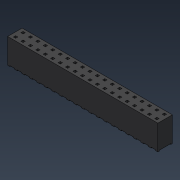
# Autodesk Inventor part: ESQ-120-33-T-D_socket
Saved by Autodesk Inventor 2022.1 (Build 261234020, 234B)
## iProperties
Created: 2017-11-11
Part Number: ESQ-120-33-T-D_socket
Catalog Web Link: www.cadenas.de
Description: ESQ Series Socket-ESQ Series - (2,54 mm) .100'' Elevated Socket
Vendor: SAMTEC
Document SubType Name: Modeling
Designer: psAdmin
Manufacturer: SAMTEC
Mass: 1.93212 g
Surface Area: 23.6719 cm^2
Volume: 1.93212 cm^3
Density: 1 g/cm^3
Material: Allgemein
Appearance: PSOLRGB-127-127-127
Category: PARTsolutions
Company: SAMTEC
PSOL_IDENT_0: {$CADENAS_DATA\23d-libs\samtec\modelling\esq\parts\esq_socket.prj},224 {VTYP=3D},{NB=ESQ-120-33-T-D_
PSOL_IDENT_1: socket},{LINA=ESQ-120-33-T-D_socket},{NN=ESQ Series Socket},{DATE=05.05.2016 11:37:34},{GEOMDATE=05.
PSOL_IDENT_2: 05.2016 11:37:00},{VERSION=},{LINEID=10},{LINESUBID=-1},{WBVAR=POS,LS,PLOPT,ROW,LLOPT,POLOPT}  {NB=E
PSOL_IDENT_3: SQ-120-33-T-D_socket},{LINA=ESQ-120-33-T-D_socket},{KT=DUMMY},{PN=ESQ-120-33-T-D},{SERIES=ESQ},{POS=
PSOL_IDENT_4: 20},{POSN=20},{POSALG=  '01','-01','02','-02','03','-03','04','-04','05','-05','06','-06','07','-07'
PSOL_IDENT_5: ,'08','-08','09','-09','10','-10','11','-11','12','-12','13','-13','14','-14','15','-15','16','-16','
PSOL_IDENT_6: 17','-17','18','-18','19','-19','20','-20','21','-21','22','-22','23','-23','24','-24','25','-25','2
PSOL_IDENT_7: 6','-26','27','-27','28','-28','29','-29','30','-30','31','-31','32','-32','33','-33','34','-34','35'
PSOL_IDENT_8: ,'-35','36','-36'  },{POSPN=20},{LS=33},{PLOPT=T},{PLOPTALG= 'G','-G = 20micro\" Selective Gold in C
PSOL_IDENT_9: ontact Area, 3micro\" Selective Gold on Tail.','T','-T = Matte Tin on Entire Pin.','S','-S =  30micr
PSOL_IDENT_10: o\" Selective Gold in Contact Area, Matte Tin on Tail.','H','-H = 30micro\" Selective Gold in Contac
PSOL_IDENT_11: t Area, 3micro\" Selective Gold on Tail.','F','-F = 3micro\" Selective Gold in Contact Area, Matte T
PSOL_IDENT_12: in on Tail.','E','-E = 50micro\" Selective Gold in Contact Area, 3micro\" Selective Gold on Tail.','
PSOL_IDENT_13: L','-L = 10micro\" Selective Gold in Contact Area, Matte Tin on Tail.' },{ROW=D},{ROWPN=-D},{ROWALG=
PSOL_IDENT_14: 'S','-S = Single Row','D','-D = Double Row','T','-T = Triple Row' },{ROWN=2},{LLOPT=},{LLOPTALG= ''
PSOL_IDENT_15: ,'Not Selected','LL','-LL = Locking Lead' },{LLOPTPN=},{POLOPT=},{POLOPTPN=},{POLOPTMAX=480},{POLOPT
PSOL_IDENT_16: MAX2='001','001','002','002','003','003','004','004','005','005','006','006','007','007','008','008'
PSOL_IDENT_17: ,'009','009','010','010','011','011','012','012','013','013','014','014','015','015','016','016','01
PSOL_IDENT_18: 7','017','018','018','019','019','020','020','021','021','022','022','023','023','024','024','025','
PSOL_IDENT_19: 025','026','026','027','027','028','028','029','029','030','030','031','031','032','032','033','033'
PSOL_IDENT_20: ,'034','034','035','035','036','036','037','037','038','038','039','039','040','040'},{POLOPTALG= ''
PSOL_IDENT_21: ,'Not Selected','001','001','002','002','003','003','004','004','005','005','006','006','007','007','
PSOL_IDENT_22: 008','008','009','009','010','010','011','011','012','012','013','013','014','014','015','015','016'
PSOL_IDENT_23: ,'016','017','017','018','018','019','019','020','020','021','021','022','022','023','023','024','02
PSOL_IDENT_24: 4','025','025','026','026','027','027','028','028','029','029','030','030','031','031','032','032','
PSOL_IDENT_25: 033','033','034','034','035','035','036','036','037','037','038','038','039','039','040','040'},{POL
PSOL_IDENT_26: ARIZE='001','001','002','002','003','003','004','004','005','005','006','006','007','007','008','008'
PSOL_IDENT_27: ,'009','009','010','010','011','011','012','012','013','013','014','014','015','015','016','016','01
PSOL_IDENT_28: 7','017','018','018','019','019','020','020','021','021','022','022','023','023','024','024','025','
PSOL_IDENT_29: 025','026','026','027','027','028','028','029','029','030','030','031','031','032','032','033','033'
PSOL_IDENT_30: ,'034','034','035','035','036','036','037','037','038','038','039','039','040','040','041','041','04
PSOL_IDENT_31: 2','042','043','043','044','044','045','045','046','046','047','047','048','048','049','049','050','
PSOL_IDENT_32: 050','051','051','052','052','053','053','054','054','055','055','056','056','057','057','058','058'
PSOL_IDENT_33: ,'059','059','060','060','061','061','062','062','063','063','064','064','065','065','066','066','06
PSOL_IDENT_34: 7','067','068','068','069','069','070','070','071','071','072','072','073','073','074','074','075','
PSOL_IDENT_35: 075','076','076','077','077','078','078','079','079','080','080','081','081','082','082','083','083'
PSOL_IDENT_36: ,'084','084','085','085','086','086','087','087','088','088','089','089','090','090','091','091','09
PSOL_IDENT_37: 2','092','093','093','094','094','095','095','096','096','097','097','098','098','099','099','100','
PSOL_IDENT_38: 100','101','101','102','102','103','103','104','104','105','105','106','106','107','107','108','108'
PSOL_IDENT_39: ,'109','109','110','110','111','111','112','112','113','113','114','114','115','115','116','116','11
PSOL_IDENT_40: 7','117','118','118','119','119','120','120','121','121','122','122','123','123','124','124','125','
PSOL_IDENT_41: 125','126','126','127','127','128','128','129','129','130','130','131','131','132','132','133','133'
PSOL_IDENT_42: ,'134','134','135','135','136','136','137','137','138','138','139','139','140','140','141','141','14
PSOL_IDENT_43: 2','142','143','143','144','144','145','145','146','146','147','147','148','148','149','149','150','
PSOL_IDENT_44: 150','151','151','152','152','153','153','154','154','155','155','156','156','157','157','158','158'
PSOL_IDENT_45: ,'159','159','160','160','161','161','162','162','163','163','164','164','165','165','166','166','16
PSOL_IDENT_46: 7','167','168','168','169','169','170','170','171','171','172','172','173','173','174','174','175','
PSOL_IDENT_47: 175','176','176','177','177','178','178','179','179','180','180','181','181','182','182','183','183'
PSOL_IDENT_48: ,'184','184','185','185','186','186','187','187','188','188','189','189','190','190','191','191','19
PSOL_IDENT_49: 2','192','193','193','194','194','195','195','196','196','197','197','198','198','199','199','200','
PSOL_IDENT_50: 200','201','201','202','202','203','203','204','204','205','205','206','206','207','207','208','208'
PSOL_IDENT_51: ,'209','209','210','210','211','211','212','212','213','213','214','214','215','215','216','216','21
PSOL_IDENT_52: 7','217','218','218','219','219','220','220','221','221','222','222','223','223','224','224','225','
PSOL_IDENT_53: 225','226','226','227','227','228','228','229','229','230','230','231','231','232','232','233','233'
PSOL_IDENT_54: ,'234','234','235','235','236','236','237','237','238','238','239','239','240','240','241','241','24
PSOL_IDENT_55: 2','242','243','243','244','244','245','245','246','246','247','247','248','248','249','249','250','
PSOL_IDENT_56: 250','251','251','252','252','253','253','254','254','255','255','256','256','257','257','258','258'
PSOL_IDENT_57: ,'259','259','260','260','261','261','262','262','263','263','264','264','265','265','266','266','26
PSOL_IDENT_58: 7','267','268','268','269','269','270','270','271','271','272','272','273','273','274','274','275','
PSOL_IDENT_59: 275','276','276','277','277','278','278','279','279','280','280','281','281','282','282','283','283'
PSOL_IDENT_60: ,'284','284','285','285','286','286','287','287','288','288','289','289','290','290','291','291','29
PSOL_IDENT_61: 2','292','293','293','294','294','295','295','296','296','297','297','298','298','299','299','300','
PSOL_IDENT_62: 300'},{POLARIZEX=0.00000},{POLARIZEY=0.00000},{POLARIZEN=0},{EVEN=0},{A=0.195},{A3DB=0.33500},{B=0.0
PSOL_IDENT_63: 9000},{C=0.635},{D=0.725},{E=0.000},{W=2.02000},{ONES=0}
NN: ESQ Series Socket
NT: ESQ Series - (2,54 mm) .100'' Elevated Socket
NB: ESQ-120-33-T-D_socket
NBSYN: $PN._socket
LINA: ESQ-120-33-T-D_socket
PN: ESQ-120-33-T-D
SERIES: ESQ
POS: -20
LS: -33
PLOPT: -T = Matte Tin on Entire Pin.
ROW: -D = Double Row
LLOPT: Not Selected
POLOPT: Not Selected
A: 0.195
SUPPLIER: SAMTEC
ARTICLENO: ESQ-120-33-T-D_socket
BOMINFO: ESQ-120-33-T-D_socket
CREATOR: CADENAS GmbH
Title: ESQ-120-33-T-D_socket
Author: Cadenas PARTsolutions
Comments: ESQ Series - (2,54 mm) .100'' Elevated Socket
Autodesk Inventor part; units mm, degrees
sketch "Sketch_1" plane through (0, 0, 0) normal (0, 1, 0) x (-1, 0, 0)
  line L0 (0, -2.4765) -> (0, 2.4765)
  line L1 (0, 2.4765) -> (-51.308, 2.4765)
  line L2 (-51.308, 2.4765) -> (-51.308, -2.4765)
  line L3 (-51.308, -2.4765) -> (0, -2.4765)
  line L4 (-49.403, 0.889) -> (-49.403, 1.651)
  line L5 (-49.403, 1.651) -> (-50.165, 1.651)
  line L6 (-50.165, 1.651) -> (-50.165, 0.889)
  line L7 (-50.165, 0.889) -> (-49.403, 0.889)
  line L8 (-49.403, -1.651) -> (-49.403, -0.889)
  line L9 (-49.403, -0.889) -> (-50.165, -0.889)
  line L10 (-50.165, -0.889) -> (-50.165, -1.651)
  line L11 (-50.165, -1.651) -> (-49.403, -1.651)
  line L12 (-46.863, 0.889) -> (-46.863, 1.651)
  line L13 (-46.863, 1.651) -> (-47.625, 1.651)
  line L14 (-47.625, 1.651) -> (-47.625, 0.889)
  line L15 (-47.625, 0.889) -> (-46.863, 0.889)
  line L16 (-46.863, -1.651) -> (-46.863, -0.889)
  line L17 (-46.863, -0.889) -> (-47.625, -0.889)
  line L18 (-47.625, -0.889) -> (-47.625, -1.651)
  line L19 (-47.625, -1.651) -> (-46.863, -1.651)
  line L20 (-44.323, 0.889) -> (-44.323, 1.651)
  line L21 (-44.323, 1.651) -> (-45.085, 1.651)
  line L22 (-45.085, 1.651) -> (-45.085, 0.889)
  line L23 (-45.085, 0.889) -> (-44.323, 0.889)
  line L24 (-44.323, -1.651) -> (-44.323, -0.889)
  line L25 (-44.323, -0.889) -> (-45.085, -0.889)
  line L26 (-45.085, -0.889) -> (-45.085, -1.651)
  line L27 (-45.085, -1.651) -> (-44.323, -1.651)
  line L28 (-41.783, 0.889) -> (-41.783, 1.651)
  line L29 (-41.783, 1.651) -> (-42.545, 1.651)
  line L30 (-42.545, 1.651) -> (-42.545, 0.889)
  line L31 (-42.545, 0.889) -> (-41.783, 0.889)
  line L32 (-41.783, -1.651) -> (-41.783, -0.889)
  line L33 (-41.783, -0.889) -> (-42.545, -0.889)
  line L34 (-42.545, -0.889) -> (-42.545, -1.651)
  line L35 (-42.545, -1.651) -> (-41.783, -1.651)
  line L36 (-39.243, 0.889) -> (-39.243, 1.651)
  line L37 (-39.243, 1.651) -> (-40.005, 1.651)
  line L38 (-40.005, 1.651) -> (-40.005, 0.889)
  line L39 (-40.005, 0.889) -> (-39.243, 0.889)
  line L40 (-39.243, -1.651) -> (-39.243, -0.889)
  line L41 (-39.243, -0.889) -> (-40.005, -0.889)
  line L42 (-40.005, -0.889) -> (-40.005, -1.651)
  line L43 (-40.005, -1.651) -> (-39.243, -1.651)
  line L44 (-36.703, 0.889) -> (-36.703, 1.651)
  line L45 (-36.703, 1.651) -> (-37.465, 1.651)
  line L46 (-37.465, 1.651) -> (-37.465, 0.889)
  line L47 (-37.465, 0.889) -> (-36.703, 0.889)
  line L48 (-36.703, -1.651) -> (-36.703, -0.889)
  line L49 (-36.703, -0.889) -> (-37.465, -0.889)
  line L50 (-37.465, -0.889) -> (-37.465, -1.651)
  line L51 (-37.465, -1.651) -> (-36.703, -1.651)
  line L52 (-34.163, 0.889) -> (-34.163, 1.651)
  line L53 (-34.163, 1.651) -> (-34.925, 1.651)
  line L54 (-34.925, 1.651) -> (-34.925, 0.889)
  line L55 (-34.925, 0.889) -> (-34.163, 0.889)
  line L56 (-34.163, -1.651) -> (-34.163, -0.889)
  line L57 (-34.163, -0.889) -> (-34.925, -0.889)
  line L58 (-34.925, -0.889) -> (-34.925, -1.651)
  line L59 (-34.925, -1.651) -> (-34.163, -1.651)
  line L60 (-31.623, 0.889) -> (-31.623, 1.651)
  line L61 (-31.623, 1.651) -> (-32.385, 1.651)
  line L62 (-32.385, 1.651) -> (-32.385, 0.889)
  line L63 (-32.385, 0.889) -> (-31.623, 0.889)
  line L64 (-31.623, -1.651) -> (-31.623, -0.889)
  line L65 (-31.623, -0.889) -> (-32.385, -0.889)
  line L66 (-32.385, -0.889) -> (-32.385, -1.651)
  line L67 (-32.385, -1.651) -> (-31.623, -1.651)
  line L68 (-29.083, 0.889) -> (-29.083, 1.651)
  line L69 (-29.083, 1.651) -> (-29.845, 1.651)
  line L70 (-29.845, 1.651) -> (-29.845, 0.889)
  line L71 (-29.845, 0.889) -> (-29.083, 0.889)
  line L72 (-29.083, -1.651) -> (-29.083, -0.889)
  line L73 (-29.083, -0.889) -> (-29.845, -0.889)
  line L74 (-29.845, -0.889) -> (-29.845, -1.651)
  line L75 (-29.845, -1.651) -> (-29.083, -1.651)
  line L76 (-26.543, 0.889) -> (-26.543, 1.651)
  line L77 (-26.543, 1.651) -> (-27.305, 1.651)
  line L78 (-27.305, 1.651) -> (-27.305, 0.889)
  line L79 (-27.305, 0.889) -> (-26.543, 0.889)
  line L80 (-26.543, -1.651) -> (-26.543, -0.889)
  line L81 (-26.543, -0.889) -> (-27.305, -0.889)
  line L82 (-27.305, -0.889) -> (-27.305, -1.651)
  line L83 (-27.305, -1.651) -> (-26.543, -1.651)
  line L84 (-24.003, 0.889) -> (-24.003, 1.651)
  line L85 (-24.003, 1.651) -> (-24.765, 1.651)
  line L86 (-24.765, 1.651) -> (-24.765, 0.889)
  line L87 (-24.765, 0.889) -> (-24.003, 0.889)
  line L88 (-24.003, -1.651) -> (-24.003, -0.889)
  line L89 (-24.003, -0.889) -> (-24.765, -0.889)
  line L90 (-24.765, -0.889) -> (-24.765, -1.651)
  line L91 (-24.765, -1.651) -> (-24.003, -1.651)
  line L92 (-21.463, 0.889) -> (-21.463, 1.651)
  line L93 (-21.463, 1.651) -> (-22.225, 1.651)
  line L94 (-22.225, 1.651) -> (-22.225, 0.889)
  line L95 (-22.225, 0.889) -> (-21.463, 0.889)
  line L96 (-21.463, -1.651) -> (-21.463, -0.889)
  line L97 (-21.463, -0.889) -> (-22.225, -0.889)
  line L98 (-22.225, -0.889) -> (-22.225, -1.651)
  line L99 (-22.225, -1.651) -> (-21.463, -1.651)
  line L100 (-18.923, 0.889) -> (-18.923, 1.651)
  line L101 (-18.923, 1.651) -> (-19.685, 1.651)
  line L102 (-19.685, 1.651) -> (-19.685, 0.889)
  line L103 (-19.685, 0.889) -> (-18.923, 0.889)
  line L104 (-18.923, -1.651) -> (-18.923, -0.889)
  line L105 (-18.923, -0.889) -> (-19.685, -0.889)
  line L106 (-19.685, -0.889) -> (-19.685, -1.651)
  line L107 (-19.685, -1.651) -> (-18.923, -1.651)
  line L108 (-16.383, 0.889) -> (-16.383, 1.651)
  line L109 (-16.383, 1.651) -> (-17.145, 1.651)
  line L110 (-17.145, 1.651) -> (-17.145, 0.889)
  line L111 (-17.145, 0.889) -> (-16.383, 0.889)
  line L112 (-16.383, -1.651) -> (-16.383, -0.889)
  line L113 (-16.383, -0.889) -> (-17.145, -0.889)
  line L114 (-17.145, -0.889) -> (-17.145, -1.651)
  line L115 (-17.145, -1.651) -> (-16.383, -1.651)
  line L116 (-13.843, 0.889) -> (-13.843, 1.651)
  line L117 (-13.843, 1.651) -> (-14.605, 1.651)
  line L118 (-14.605, 1.651) -> (-14.605, 0.889)
  line L119 (-14.605, 0.889) -> (-13.843, 0.889)
  line L120 (-13.843, -1.651) -> (-13.843, -0.889)
  line L121 (-13.843, -0.889) -> (-14.605, -0.889)
  line L122 (-14.605, -0.889) -> (-14.605, -1.651)
  line L123 (-14.605, -1.651) -> (-13.843, -1.651)
  line L124 (-11.303, 0.889) -> (-11.303, 1.651)
  line L125 (-11.303, 1.651) -> (-12.065, 1.651)
  line L126 (-12.065, 1.651) -> (-12.065, 0.889)
  line L127 (-12.065, 0.889) -> (-11.303, 0.889)
  line L128 (-11.303, -1.651) -> (-11.303, -0.889)
  line L129 (-11.303, -0.889) -> (-12.065, -0.889)
  line L130 (-12.065, -0.889) -> (-12.065, -1.651)
  line L131 (-12.065, -1.651) -> (-11.303, -1.651)
  line L132 (-8.763, 0.889) -> (-8.763, 1.651)
  line L133 (-8.763, 1.651) -> (-9.525, 1.651)
  line L134 (-9.525, 1.651) -> (-9.525, 0.889)
  line L135 (-9.525, 0.889) -> (-8.763, 0.889)
  line L136 (-8.763, -1.651) -> (-8.763, -0.889)
  line L137 (-8.763, -0.889) -> (-9.525, -0.889)
  line L138 (-9.525, -0.889) -> (-9.525, -1.651)
  line L139 (-9.525, -1.651) -> (-8.763, -1.651)
  line L140 (-6.223, 0.889) -> (-6.223, 1.651)
  line L141 (-6.223, 1.651) -> (-6.985, 1.651)
  line L142 (-6.985, 1.651) -> (-6.985, 0.889)
  line L143 (-6.985, 0.889) -> (-6.223, 0.889)
  line L144 (-6.223, -1.651) -> (-6.223, -0.889)
  line L145 (-6.223, -0.889) -> (-6.985, -0.889)
  line L146 (-6.985, -0.889) -> (-6.985, -1.651)
  line L147 (-6.985, -1.651) -> (-6.223, -1.651)
  line L148 (-3.683, 0.889) -> (-3.683, 1.651)
  line L149 (-3.683, 1.651) -> (-4.445, 1.651)
  line L150 (-4.445, 1.651) -> (-4.445, 0.889)
  line L151 (-4.445, 0.889) -> (-3.683, 0.889)
  line L152 (-3.683, -1.651) -> (-3.683, -0.889)
  line L153 (-3.683, -0.889) -> (-4.445, -0.889)
  line L154 (-4.445, -0.889) -> (-4.445, -1.651)
  line L155 (-4.445, -1.651) -> (-3.683, -1.651)
  line L156 (-1.143, 0.889) -> (-1.143, 1.651)
  line L157 (-1.143, 1.651) -> (-1.905, 1.651)
  line L158 (-1.905, 1.651) -> (-1.905, 0.889)
  line L159 (-1.905, 0.889) -> (-1.143, 0.889)
  line L160 (-1.143, -1.651) -> (-1.143, -0.889)
  line L161 (-1.143, -0.889) -> (-1.905, -0.889)
  line L162 (-1.905, -0.889) -> (-1.905, -1.651)
  line L163 (-1.905, -1.651) -> (-1.143, -1.651)
  constraints: 328 end point
extrude "Extrusion1" add sketch "Sketch_1" along normal blind 8.509
sketch "Sketch_2" plane through (0, 0, 0) normal (0, 1, 0) x (-1, 0, 0)
  line L0 (0, -2.4765) -> (0, 2.4765)
  line L1 (0, 2.4765) -> (-51.308, 2.4765)
  line L2 (-51.308, 2.4765) -> (-51.308, -2.4765)
  line L3 (-51.308, -2.4765) -> (0, -2.4765)
  constraints: 8 end point
extrude "Extrusion2" add sketch "Sketch_2" along normal blind 1.143
sketch "Sketch_9" plane through (0, 0, 0) normal (1, 0, 0) x (0, 1, 0)
  line L0 (0.254, 1.9685) -> (0, 1.9685)
  line L1 (0, 1.9685) -> (0, -1.9685)
  line L2 (0, -1.9685) -> (0.254, -1.9685)
  line L3 (0.254, -1.9685) -> (0.254, 1.9685)
  constraints: 8 end point
extrude "Extrusion3" cut sketch "Sketch_9" along normal blind 51.308
sketch "Sketch_11" plane through (0, 0, 0) normal (0, 0, 1) x (1, 0, 0)
  line L0 (0.254, 0) -> (0.254, -1.27)
  line L1 (0.254, -1.27) -> (51.562, -1.27)
  line L2 (51.562, -1.27) -> (51.562, 0)
  line L3 (51.562, 0) -> (50.546, 0)
  line L4 (50.546, 0) -> (50.546, 0.254)
  line L5 (50.546, 0.254) -> (49.022, 0.254)
  line L6 (49.022, 0.254) -> (49.022, 0)
  line L7 (49.022, 0) -> (48.006, 0)
  line L8 (48.006, 0) -> (48.006, 0.254)
  line L9 (48.006, 0.254) -> (46.482, 0.254)
  line L10 (46.482, 0.254) -> (46.482, 0)
  line L11 (46.482, 0) -> (45.466, 0)
  line L12 (45.466, 0) -> (45.466, 0.254)
  line L13 (45.466, 0.254) -> (43.942, 0.254)
  line L14 (43.942, 0.254) -> (43.942, 0)
  line L15 (43.942, 0) -> (42.926, 0)
  line L16 (42.926, 0) -> (42.926, 0.254)
  line L17 (42.926, 0.254) -> (41.402, 0.254)
  line L18 (41.402, 0.254) -> (41.402, 0)
  line L19 (41.402, 0) -> (40.386, 0)
  line L20 (40.386, 0) -> (40.386, 0.254)
  line L21 (40.386, 0.254) -> (38.862, 0.254)
  line L22 (38.862, 0.254) -> (38.862, 0)
  line L23 (38.862, 0) -> (37.846, 0)
  line L24 (37.846, 0) -> (37.846, 0.254)
  line L25 (37.846, 0.254) -> (36.322, 0.254)
  line L26 (36.322, 0.254) -> (36.322, 0)
  line L27 (36.322, 0) -> (35.306, 0)
  line L28 (35.306, 0) -> (35.306, 0.254)
  line L29 (35.306, 0.254) -> (33.782, 0.254)
  line L30 (33.782, 0.254) -> (33.782, 0)
  line L31 (33.782, 0) -> (32.766, 0)
  line L32 (32.766, 0) -> (32.766, 0.254)
  line L33 (32.766, 0.254) -> (31.242, 0.254)
  line L34 (31.242, 0.254) -> (31.242, 0)
  line L35 (31.242, 0) -> (30.226, 0)
  line L36 (30.226, 0) -> (30.226, 0.254)
  line L37 (30.226, 0.254) -> (28.702, 0.254)
  line L38 (28.702, 0.254) -> (28.702, 0)
  line L39 (28.702, 0) -> (27.686, 0)
  line L40 (27.686, 0) -> (27.686, 0.254)
  line L41 (27.686, 0.254) -> (26.162, 0.254)
  line L42 (26.162, 0.254) -> (26.162, 0)
  line L43 (26.162, 0) -> (25.146, 0)
  line L44 (25.146, 0) -> (25.146, 0.254)
  line L45 (25.146, 0.254) -> (23.622, 0.254)
  line L46 (23.622, 0.254) -> (23.622, 0)
  line L47 (23.622, 0) -> (22.606, 0)
  line L48 (22.606, 0) -> (22.606, 0.254)
  line L49 (22.606, 0.254) -> (21.082, 0.254)
  line L50 (21.082, 0.254) -> (21.082, 0)
  line L51 (21.082, 0) -> (20.066, 0)
  line L52 (20.066, 0) -> (20.066, 0.254)
  line L53 (20.066, 0.254) -> (18.542, 0.254)
  line L54 (18.542, 0.254) -> (18.542, 0)
  line L55 (18.542, 0) -> (17.526, 0)
  line L56 (17.526, 0) -> (17.526, 0.254)
  line L57 (17.526, 0.254) -> (16.002, 0.254)
  line L58 (16.002, 0.254) -> (16.002, 0)
  line L59 (16.002, 0) -> (14.986, 0)
  line L60 (14.986, 0) -> (14.986, 0.254)
  line L61 (14.986, 0.254) -> (13.462, 0.254)
  line L62 (13.462, 0.254) -> (13.462, 0)
  line L63 (13.462, 0) -> (12.446, 0)
  line L64 (12.446, 0) -> (12.446, 0.254)
  line L65 (12.446, 0.254) -> (10.922, 0.254)
  line L66 (10.922, 0.254) -> (10.922, 0)
  line L67 (10.922, 0) -> (9.906, 0)
  line L68 (9.906, 0) -> (9.906, 0.254)
  line L69 (9.906, 0.254) -> (8.382, 0.254)
  line L70 (8.382, 0.254) -> (8.382, 0)
  line L71 (8.382, 0) -> (7.366, 0)
  line L72 (7.366, 0) -> (7.366, 0.254)
  line L73 (7.366, 0.254) -> (5.842, 0.254)
  line L74 (5.842, 0.254) -> (5.842, 0)
  line L75 (5.842, 0) -> (4.826, 0)
  line L76 (4.826, 0) -> (4.826, 0.254)
  line L77 (4.826, 0.254) -> (3.302, 0.254)
  line L78 (3.302, 0.254) -> (3.302, 0)
  line L79 (3.302, 0) -> (2.286, 0)
  line L80 (2.286, 0) -> (2.286, 0.254)
  line L81 (2.286, 0.254) -> (0.762, 0.254)
  line L82 (0.762, 0.254) -> (0.762, 0)
  line L83 (0.762, 0) -> (0.254, 0)
  constraints: 168 end point
extrude "Extrusion4" cut sketch "Sketch_11" along normal mid plane 4.953
ref_plane "socket_XY" through (25.654, 0, 0) normal (0, 1, 0) x (1, 0, 0)
ref_plane "socket_YZ" through (25.654, 0, 0) normal (1, 0, 0) x (0, 0, -1)
ref_plane "socket_ZX" through (25.654, 0, 0) normal (0, 0, -1) x (0, 1, 0)
ref_plane "to_bottom_socket_XY" through (25.654, -7.62, 0) normal (0, 1, 0) x (1, 0, 0)
ref_plane "to_bottom_socket_YZ" through (25.654, -7.62, 0) normal (1, 0, 0) x (0, 0, -1)
ref_plane "to_bottom_socket_ZX" through (25.654, -7.62, 0) normal (0, 0, -1) x (0, 1, 0)
body "Solid1"
